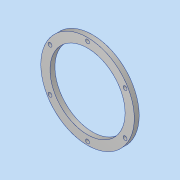
# Autodesk Inventor part: AluminumSealingDisc
Saved by Autodesk Inventor 2017 (Build 210142000, 142)
## iProperties
Created: 2016-10-25
Part Number: AluminumSealingDisc
Material: Aluminum 6061
Document SubType Name: Modeling
Designer: techn
Density: 2.7 g/cm^3
Appearance: Aluminum - Flat
Mass: 28.6556 g
Surface Area: 71.8195 cm^2
Volume: 10.6132 cm^3
Author: techn
Autodesk Inventor part; units mm, degrees
ref_plane "YZ Plane" through (0, 0, 0) normal (1, 0, 0) x (0, 1, 0)
ref_plane "XZ Plane" through (0, 0, 0) normal (0, 1, 0) x (-1, 0, 0)
ref_plane "XY Plane" through (0, 0, 0) normal (0, 0, 1) x (1, 0, 0)
sketch "Sketch1" plane through (0, 0, 0) normal (0, 0, 1) x (1, 0, 0)
  circle A0 centre (0, 0) radius 45.212
  dimension "d0" = 90.424
  constraints: 1 centre point, 1 coincident
  measures "d0" diameter of A0
extrude "Extrusion1" add sketch "Sketch1" along normal blind 4.7625
sketch "Sketch2" plane through (0, 0, 0) normal (0, 0, -1) x (-1, 0, 0)
  circle A0 centre (0, 0) radius 25.4
  dimension "d3" = 50.8
  constraints: 1 centre point, 1 coincident
  measures "d3" diameter of A0
extrude "Extrusion2" cut sketch "Sketch2" against normal blind 4.7625
sketch "Sketch4" plane through (0, 0, 4.7625) normal (0, 0, 1) x (1, 0, 0)
  circle A0 centre (0, 41.91) radius 1.905
  circle A1 centre (-36.2951, 20.955) radius 1.905
  circle A2 centre (-36.2951, -20.955) radius 1.905
  circle A3 centre (0, -41.91) radius 1.905
  circle A4 centre (36.2951, -20.955) radius 1.905
  circle A5 centre (36.2951, 20.955) radius 1.905
  point P0 (0, 0)
  dimension "d14" = 3.81
  dimension "d15" = 41.91
  dimension "d18" = 360
  constraints: 6 centre point, 13 other
  measures "d14" diameter of A0
  measures "d15" distance of A0.centre point (0, 0)
extrude "Extrusion4" cut sketch "Sketch4" against normal blind 25.4
sketch "Sketch5" plane through (0, 0, 4.7625) normal (0, 0, 1) x (1, 0, 0)
  circle A0 centre (20.795, 25.8191) radius 3.175
  line L0 (0, 0) -> (0, 18.2107)
  circle A1 centre (-20.795, 25.8191) radius 3.175
  dimension "d22" = 6.35
  dimension "d23" = 25.8191
  dimension "d24" = 20.795
  constraints: 2 centre point, 2 end point, 1 symmetric about line, 1 vertical, 1 other
  measures "d22" diameter of A0
  measures "d23" vertical distance of A0.centre L0.start
  measures "d24" horizontal distance of A0.centre L0.start
extrude "Extrusion5" cut sketch "Sketch5" against normal blind 25.4
sketch "Sketch6" plane through (0, 0, 4.7625) normal (0, 0, 1) x (1, 0, 0)
  circle A0 centre (20.795, 25.8191) radius 3.175 projected
  circle A1 centre (-20.795, 25.8191) radius 3.175 projected
  circle A2 centre (36.2951, -20.955) radius 1.905 projected
  circle A3 centre (-36.2951, -20.955) radius 1.905 projected
  circle A4 centre (0, 41.91) radius 1.905 projected
  circle A5 centre (-36.2951, 20.955) radius 1.905 projected
  circle A6 centre (0, -41.91) radius 1.905 projected
  circle A7 centre (36.2951, 20.955) radius 1.905 projected
  circle A8 centre (0, 0) radius 25.4 projected
  circle A9 centre (0, 0) radius 45.212 projected
  circle A10 centre (0, 0) radius 36.327
  circle A11 centre (-20.795, 25.8191) radius 3.175 projected
  constraints: 1 centre point, 1 coincident, 1 tangent
extrude "Extrusion6" cut sketch "Sketch6" against normal blind 25.4 contours A10
body "Solid1"
